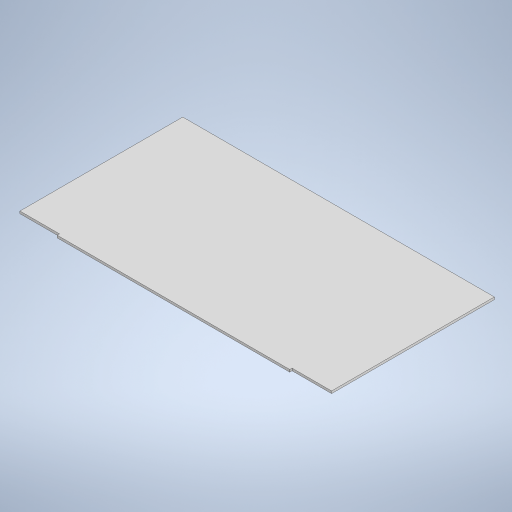
# Autodesk Inventor part: Base Plate Wall 1
Saved by Autodesk Inventor 2023 (Build 270158000, 158)
## iProperties
Created: 2023-02-07
Part Number: Base Plate Wall 1
Material: Generic
Document SubType Name: Modeling
Designer: cheng
Density: 1 g/cm^3
Appearance: Default
Author: cheng
Autodesk Inventor part; units mm, degrees
ref_plane "YZ Plane" through (0, 0, 0) normal (1, 0, 0) x (0, 1, 0)
ref_plane "XZ Plane" through (0, 0, 0) normal (0, 1, 0) x (-1, 0, 0)
ref_plane "XY Plane" through (0, 0, 0) normal (0, 0, 1) x (1, 0, 0)
sketch "Sketch1" plane through (0, 0, 0) normal (0, 1, 0) x (-1, 0, 0)
  line L0 (335, -175) -> (-335, -175)
  line L1 (-335, -175) -> (-335, 175)
  line L2 (-335, 175) -> (335, 175)
  line L3 (335, 175) -> (335, -175)
  line L4 (335, -175) -> (-335, 175) construction
  line L5 (-335, -175) -> (335, 175) construction
  line L6 (-250, 180) -> (250, 180)
  line L7 (250, 180) -> (250, 175)
  line L8 (250, 175) -> (-250, 175)
  line L9 (-250, 175) -> (-250, 180)
  line L10 (-250, 180) -> (250, 175) construction
  line L11 (250, 180) -> (-250, 175) construction
  line L12 (0, -175) -> (0, 177.5) construction
  line L13 (0, 175) -> (0, 180) construction
  line L14 (335, -133.7323) -> (340, -133.7323)
  line L15 (340, -133.7323) -> (340, 136.2323)
  line L16 (340, 136.2323) -> (335, 136.2323)
  line L17 (335, 136.2323) -> (335, -133.7323)
  line L18 (335, -133.7323) -> (340, 136.2323) construction
  line L19 (340, -133.7323) -> (335, 136.2323) construction
  point P0 (0, 0)
  point P1 (0, 177.5)
  point P2 (250, 175)
  point P3 (-250, 175)
  point P4 (337.5, 1.25)
  dimension "d2" = 5
  dimension "d3" = 670
  dimension "d4" = 500
  dimension "d5" = 350
  dimension "d9" = 5
  constraints: 40 end point, 10 midpoint, 6 parallel, 4 perpendicular, 3 collinear, 3 horizontal
  measures "d2" distance of L8.end L6.start
  measures "d3" distance of L0.start L0.end
  measures "d4" distance of L6.start L6.end
  measures "d5" distance between parallel lines of L2 L0
  measures "d9" distance between parallel lines of L15 L17
extrude "Extrusion1" add sketch "Sketch1" along normal blind 5 contours L0 L1 L2 L3 | L9 L6 L7 L2
body "Solid1"
